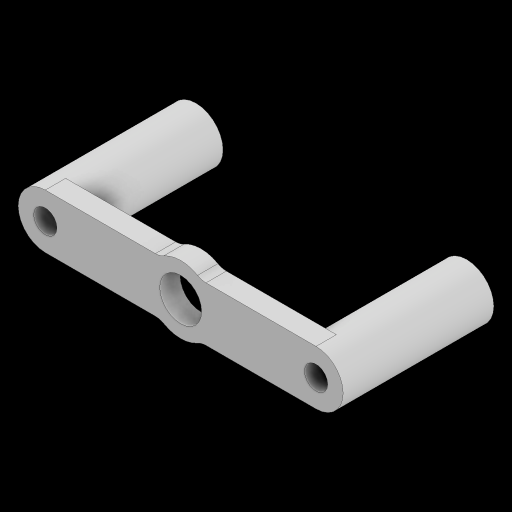
# Autodesk Inventor part: DrivenHolder
Saved by Autodesk Inventor 2024.1 (Build 281209000, 209)
## iProperties
Created: 2025-05-08
Part Number: DrivenHolder
Material: Generic
Document SubType Name: Modeling
Designer: Teddy
Density: 1 g/cm^3
Appearance: Default
Author: Teddy
Autodesk Inventor part; units mm, degrees
ref_plane "Work Plane1" through (0, 0, 0) normal (0, 0, 1) x (1, 0, 0)
sketch "Sketch1" plane through (0, 0, 0) normal (0, 0, 1) x (1, 0, 0)
  circle A0 centre (0, -16.9188) radius 2.1844 projected
  circle A1 centre (-25.4, -16.9188) radius 2.1844 projected
  circle A2 centre (25.4, -16.9188) radius 2.1844 projected
  circle A3 centre (-25.4, -16.9188) radius 5.08
  circle A4 centre (25.4, -16.9188) radius 5.08
  circle A5 centre (0, -16.9188) radius 3.937
  arc A6 (-3.81, -21.9988) -> (3.81, -21.9988) centre (0, -16.9188) ccw
  arc A7 (3.81, -11.8388) -> (-3.81, -11.8388) centre (0, -16.9188) ccw
  line L0 (-25.4, -11.8388) -> (-3.81, -11.8388)
  line L1 (3.81, -11.8388) -> (25.4, -11.8388)
  line L2 (25.4, -21.9988) -> (3.81, -21.9988)
  line L3 (-3.81, -21.9988) -> (-25.4, -21.9988)
  point P0 (0, 0)
  dimension "d0" = 10.16
  dimension "d1" = 10.16
  dimension "d2" = 7.874
  constraints: 8 end point, 8 point on circle, 8 tangent, 5 centre point, 4 coincident
  measures "d0" diameter of A3
  measures "d1" diameter of A4
  measures "d2" diameter of A5
extrude "Extrusion1" add sketch "Sketch1" along normal blind 3.81 contours A3 | A3 L0 A7 L1 A4 L2 A6 L3 | A4
fillet "Fillet1" radius 3.175 4 edges at (-3.81, -11.8388, 1.905) (3.81, -11.8388, 1.905) (3.81, -21.9988, 1.905) (-3.81, -21.9988, 1.905)
sketch "Sketch3" plane through (0, 0, 0) normal (0, 0, -1) x (-1, 0, 0)
  circle A0 centre (25.4, -16.9188) radius 5.08 projected
  circle A1 centre (25.4, -16.9188) radius 2.1844 projected
  arc A2 (25.4, -21.9988) -> (25.4, -11.8388) centre (25.4, -16.9188) ccw projected
  circle A3 centre (-25.4, -16.9188) radius 5.08 projected
  circle A4 centre (-25.4, -16.9188) radius 2.1844 projected
  point P0 (0, 0)
ref_plane "Work Plane2" through (-114.3, -27.2375, -10.16) normal (0, 0, 1) x (1, 0, 0)
ref_plane "Work Plane3" through (-101.6, -27.4915, -24.4475) normal (0, 0, 1) x (1, 0, 0)
extrude "Extrusion2" add sketch "Sketch3" along normal up to surface (24.4475 mm away)
body "Solid1"
